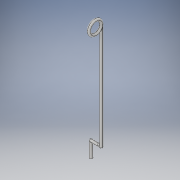
# Autodesk Inventor part: rod
Saved by Autodesk Inventor 2017 (Build 210142000, 142)
## iProperties
Created: 2016-12-13
Part Number: rod
Material: Generic
Document SubType Name: Modeling
Designer: PLTW
Density: 1 g/cm^3
Appearance: Default
Author: PLTW
Autodesk Inventor part; units mm, degrees
ref_plane "YZ Plane" through (0, 0, 0) normal (1, 0, 0) x (0, 1, 0)
ref_plane "XZ Plane" through (0, 0, 0) normal (0, 1, 0) x (-1, 0, 0)
ref_plane "XY Plane" through (0, 0, 0) normal (0, 0, 1) x (1, 0, 0)
sketch "Sketch1" plane through (0, 0, 0) normal (0, 0, 1) x (1, 0, 0)
  line L0 (0, 0) -> (0, 4.9022)
  line L1 (0, 4.9022) -> (3.048, 4.9022)
  line L2 (3.048, 4.9022) -> (3.048, 36.0934)
  line L3 (3.048, 36.0934) -> (3.9116, 36.0934)
  line L4 (3.9116, 36.0934) -> (3.9116, 4.0386)
  line L5 (3.9116, 4.0386) -> (0.8636, 4.0386)
  line L6 (0.8636, 4.0386) -> (0.8636, 0)
  line L7 (0.8636, 0) -> (0, 0)
  dimension "d4" = 3.9116
  dimension "d5" = 4.9022
  dimension "d6" = 32.0548
  dimension "d9" = 0.8636
  dimension "d10" = 0.8636
  dimension "d11" = 0.8636
  constraints: 16 end point, 7 perpendicular, 1 vertical
  measures "d4" distance between parallel lines of L4 L0
  measures "d5" distance between parallel lines of L7 L1
  measures "d6" distance of L3.end L4.end
  measures "d9" distance of L6.end L0.start
  measures "d10" distance between parallel lines of L1 L5
  measures "d11" distance between parallel lines of L2 L4
extrude "Extrusion1" add sketch "Sketch1" along normal blind 0.8636
sketch "Sketch2" plane through (3.9116, 4.0386, 0) normal (1, 0, 0) x (0, 0, -1)
  line L0 (0, 0.8636) -> (0, 32.0548) projected
  line L1 (-0.8636, 0) -> (-0.8636, 32.0548) projected
  circle A0 centre (-2.2606, 32.0548) radius 1.397
  circle A1 centre (-2.2606, 32.0548) radius 2.2606
  point P0 (0, -4.0386)
  dimension "d12" = 2.794
  constraints: 1 centre point, 1 coincident, 1 horizontal alignment, 1 tangent, 1 vertical, 2 other
  measures "d12" diameter of A0
extrude "Extrusion3" add sketch "Sketch2" against normal up to surface (0.8636 mm away)
fillet "Fillet1" radius 0.4191 19 edges at (3.9116, 37.0814, 4.2939) (3.9116, 20.066, 0) (3.048, 37.0814, 4.2939) (3.048, 20.4978, 0) (3.9116, 19.1774, 0.8636) (3.048, 19.6092, 0.8636) (1.524, 4.9022, 0) (2.3876, 4.0386, 0) (1.524, 4.9022, 0.8636) (0.8636, 2.0193, 0) (0, 2.4511, 0) (0.8636, 2.0193, 0.8636) (0, 2.4511, 0.8636) (2.3876, 4.0386, 0.8636) (0, 4.9022, 0.4318) (3.9116, 4.0386, 0.4318) (3.048, 4.9022, 0.4318) (3.9116, 36.0934, 3.6576) (3.048, 36.0934, 3.6576)
equation "\"d10\" = d9"
equation "\"d11\" = d9"
body "Solid1"
